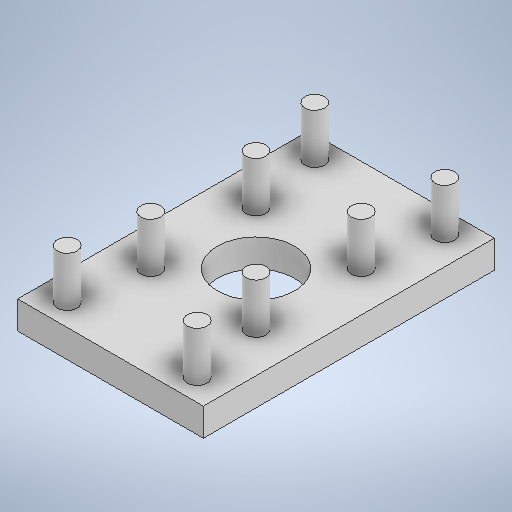
# Autodesk Inventor part: Plate2
Saved by Autodesk Inventor 2027 (Build 310192060, 192F)
## iProperties
Created: 2026-07-07
Part Number: Plate2
Material: Generic
Document SubType Name: Modeling
Designer: 13129
Density: 1 g/cm^3
Appearance: Default
Author: 13129
Autodesk Inventor part; units mm, degrees
ref_plane "YZ Plane" through (0, 0, 0) normal (1, 0, 0) x (0, 1, 0)
ref_plane "XZ Plane" through (0, 0, 0) normal (0, 1, 0) x (-1, 0, 0)
ref_plane "XY Plane" through (0, 0, 0) normal (0, 0, 1) x (1, 0, 0)
sketch "Sketch1" plane through (0, 0, 0) normal (0, 1, 0) x (-1, 0, 0)
  line L0 (0, 0) -> (0, -47)
  line L1 (0, -47) -> (30, -47)
  line L2 (30, -47) -> (30, 0)
  line L3 (30, 0) -> (0, 0)
  circle A0 centre (15, -23.5) radius 6.25
  circle A1 centre (6.5, -32) radius 1.6
  circle A2 centre (23.5, -32) radius 1.6
  circle A3 centre (25.5, -43.5) radius 1.6
  circle A4 centre (4.5, -43.5) radius 1.6
  circle A5 centre (6.5, -15) radius 1.6
  circle A6 centre (23.5, -15) radius 1.6
  circle A7 centre (25.5, -3.5) radius 1.6
  circle A8 centre (4.5, -3.5) radius 1.6
  line L4 (23.5, -32) -> (6.5, -32)
  line L5 (6.5, -32) -> (6.5, -15)
  line L6 (25.5, -43.5) -> (4.5, -43.5)
  line L7 (4.5, -43.5) -> (4.5, -3.5)
  point P0 (30, -23.5)
  point P1 (15, -47)
  point P2 (4.5, -23.5)
  point P3 (0, -23.5)
  point P4 (15, -43.5)
  point P5 (15, -32)
  point P6 (15, 0)
  point P7 (6.5, -23.5)
  dimension "d0" = 47
  dimension "d1" = 30
  dimension "d2" = 3.2
  dimension "d3" = 12.5
  dimension "d4" = 40
  dimension "d5" = 21
  dimension "d6" = 17
  dimension "d7" = 17
  constraints: 16 end point, 9 centre point, 8 midpoint, 7 equal radius, 7 horizontal alignment, 7 vertical alignment, 5 perpendicular, 2 horizontal, 1 vertical
  measures "d0" distance of L0.start L0.end
  measures "d1" distance of L0.end L1.end
  measures "d2" diameter of A3
  measures "d3" diameter of A0
  measures "d4" distance of L6.end L7.end
  measures "d5" distance of L6.start L6.end
  measures "d6" distance of L4.end L5.end
  measures "d7" distance of L4.start L4.end
extrude "Extrusion1" add sketch "Sketch1" along normal blind 4.5
sketch "Sketch2" plane through (0, 0, 0) normal (0, -1, 0) x (1, 0, 0)
  circle A0 centre (-4.5, -3.5) radius 1.6 construction
  circle A1 centre (-4.5, -43.5) radius 1.6 construction
  circle A2 centre (-6.5, -15) radius 1.6 construction
  circle A3 centre (-23.5, -32) radius 1.6 construction
  circle A4 centre (-6.5, -32) radius 1.6 construction
  circle A5 centre (-25.5, -43.5) radius 1.6 construction
  circle A6 centre (-23.5, -15) radius 1.6 construction
  circle A7 centre (-25.5, -3.5) radius 1.6 construction
  circle A8 centre (-25.5, -43.5) radius 1.6
  circle A9 centre (-4.5, -43.5) radius 1.6
  circle A10 centre (-6.5, -32) radius 1.6
  circle A11 centre (-6.5, -15) radius 1.6
  circle A12 centre (-4.5, -3.5) radius 1.6
  circle A13 centre (-25.5, -3.5) radius 1.6
  circle A14 centre (-23.5, -15) radius 1.6
  circle A15 centre (-23.5, -32) radius 1.6
  constraints: 8 centre point, 8 coincident, 8 concentric
extrude "Extrusion2" add sketch "Sketch2" against normal blind 12.5
body "Solid1"
